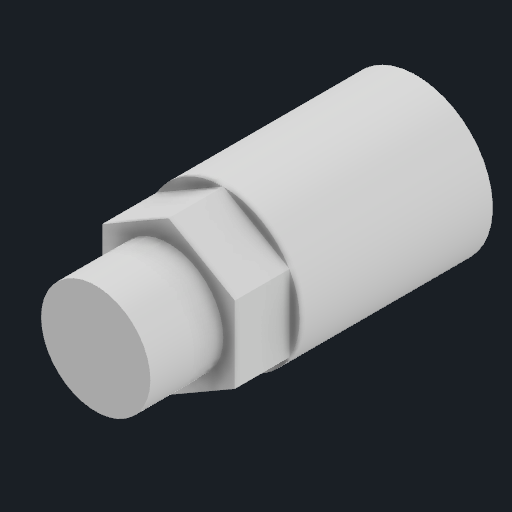
# Autodesk Inventor part: pm6m6 fitting dtraight
Saved by Autodesk Inventor 2024.3 (Build 283343000, 343)
## iProperties
Created: 2024-11-28
Part Number: pm6m6 fitting dtraight
Material: Generic
Document SubType Name: Modeling
Designer: MFil
Density: 7.15978 g/cm^3
Appearance: Default
Mass: 6 g
Surface Area: 5.41561 cm^2
Volume: 0.838015 cm^3
Author: MFil
Autodesk Inventor part; units mm, degrees
ref_plane "YZ Plane" through (0, 0, 0) normal (1, 0, 0) x (0, 1, 0)
ref_plane "XZ Plane" through (0, 0, 0) normal (0, 1, 0) x (-1, 0, 0)
ref_plane "XY Plane" through (0, 0, 0) normal (0, 0, 1) x (1, 0, 0)
sketch "Sketch1" plane through (0, 0, 0) normal (0, 1, 0) x (-1, 0, 0)
  line L0 (24, -38) -> (28.2, -38)
  line L1 (28.2, -38) -> (28.2, -55.6)
  line L2 (28.2, -55.6) -> (24, -55.6)
  line L3 (24, -55.6) -> (24, -38)
  line L4 (24, -38) -> (27, -38)
  line L5 (27, -38) -> (27, -42)
  line L6 (27, -42) -> (24, -42)
  line L7 (24, -42) -> (24, -38)
  line L8 (27, -42) -> (28.2, -42)
  line L9 (28.2, -42) -> (28.2, -38)
  line L10 (28.2, -38) -> (27, -38)
  line L11 (27, -38) -> (27, -42)
  point P0 (0, 0)
  dimension "d0" = 4.2
  dimension "d1" = 17.6
  dimension "d2" = 3
  dimension "d3" = 4
  constraints: 24 end point, 6 parallel, 3 horizontal, 3 perpendicular
  measures "d0" distance of L1.end L2.end
  measures "d1" distance of L0.end L1.end
  measures "d2" distance of L5.end L6.end
  measures "d3" distance of L4.end L5.end
revolve "Revolution1" add sketch "Sketch1" angle 360 about axis through (-24, 0, -55.6) along (0, 0, 1) contours L0 L5 L6 L3 | L6 L8 L1 L2 L3
sketch "Sketch2" plane through (-24, 0, -42) normal (0, 0, 1) x (1, 0, 0)
  circle A0 centre (0, 0) radius 3 projected
  circle A1 centre (0, 0) radius 4.2 projected
  line L0 (0, 4.2) -> (3.6373, 2.1)
  line L1 (3.6373, 2.1) -> (3.6373, -2.1)
  line L2 (3.6373, -2.1) -> (0, -4.2)
  line L3 (0, -4.2) -> (-3.6373, -2.1)
  line L4 (-3.6373, -2.1) -> (-3.6373, 2.1)
  line L5 (-3.6373, 2.1) -> (0, 4.2)
  point P0 (24, 0)
  point P1 (-3.6373, 2.1)
  point P2 (-3.6373, 2.1)
  point P3 (-3.6373, -2.1)
  point P4 (-3.6373, -2.1)
  point P5 (0, -4.2)
  point P6 (0, -4.2)
  point P7 (3.6373, 2.1)
  point P8 (3.6373, 2.1)
  constraints: 12 end point, 1 coincident, 15 other
extrude "Extrusion1" cut sketch "Sketch2" against normal blind 3 contours A1 L1 | L0 A1 | A1 L2 | L5 A1 | A1 L3 | L4 A1
body "Solid1"
